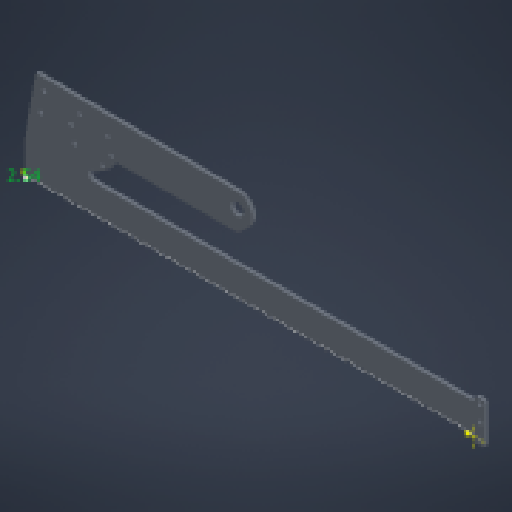
# Autodesk Inventor part: RACK_LINEARINTAKE
Saved by Autodesk Inventor 2026.2 (Build 302298010, 298A)
## iProperties
Created: 2026-04-01
Part Number: RACK_LINEARINTAKE
Material: Polycarbonate, RcM70, Black
Document SubType Name: Modeling
Designer: 4aida
Density: 11.9024 g/cm^3
Appearance: Grey (Dark)
Author: 4aida
Autodesk Inventor part; units mm, degrees
(part 1 of 2)
ref_plane "YZ Plane" through (0, 0, 0) normal (1, 0, 0) x (0, 1, 0)
ref_plane "XZ Plane" through (0, 0, 0) normal (0, 1, 0) x (-1, 0, 0)
ref_plane "XY Plane" through (0, 0, 0) normal (0, 0, 1) x (1, 0, 0)
sketch "Sketch1" plane through (0, 0, 0) normal (0, 0, 1) x (1, 0, 0)
  line L0 (7.1726, 5.588) -> (5.2604, 0.3343)
  arc A0 (4.783, 0) -> (5.2604, 0.3343) centre (4.783, 0.508) ccw
  line L1 (4.783, 0) -> (3.1966, 0)
  arc A1 (2.7192, 0.3343) -> (3.1966, 0) centre (3.1966, 0.508) ccw
  line L2 (2.7192, 0.3343) -> (0.807, 5.588)
  line L3 (-0.807, 5.588) -> (0.807, 5.588)
  line L4 (-0.807, 5.588) -> (-2.7192, 0.3343)
  arc A2 (-3.1966, 0) -> (-2.7192, 0.3343) centre (-3.1966, 0.508) ccw
  line L5 (-3.1966, 0) -> (-4.783, 0)
  arc A3 (-5.2604, 0.3343) -> (-4.783, 0) centre (-4.783, 0.508) ccw
  line L6 (-5.2604, 0.3343) -> (-7.1726, 5.588)
  line L7 (-3.9898, 0) -> (3.9898, 0) construction
  line L8 (7.1726, 27.5119) -> (7.1726, 38.1)
  line L9 (7.1726, 38.1) -> (-557.7681, 38.1)
  line L10 (-557.7681, 38.1) -> (-557.7681, 5.588)
  line L11 (-5.2604, 0.3343) -> (-7.1726, 5.588)
  line L12 (-11.9695, 0) -> (-3.9898, 0) construction
  line L13 (-8.7867, 5.588) -> (-10.6989, 0.3343)
  arc A4 (-11.1763, 0) -> (-10.6989, 0.3343) centre (-11.1763, 0.508) ccw
  line L14 (-11.1763, 0) -> (-12.7627, 0)
  arc A5 (-13.24, 0.3343) -> (-12.7627, 0) centre (-12.7627, 0.508) ccw
  line L15 (-13.24, 0.3343) -> (-15.1523, 5.588)
  arc A6 (-5.2604, 0.3343) -> (-4.783, 0) centre (-4.783, 0.508) ccw
  line L16 (-3.1966, 0) -> (-4.783, 0)
  arc A7 (-3.1966, 0) -> (-2.7192, 0.3343) centre (-3.1966, 0.508) ccw
  line L17 (-0.807, 5.588) -> (-2.7192, 0.3343)
  line L18 (-8.7867, 5.588) -> (-7.1726, 5.588)
  line L19 (-13.24, 0.3343) -> (-15.1523, 5.588)
  line L20 (-19.9491, 0) -> (-11.9695, 0) construction
  line L21 (-16.7663, 5.588) -> (-18.6785, 0.3343)
  arc A8 (-19.1559, 0) -> (-18.6785, 0.3343) centre (-19.1559, 0.508) ccw
  line L22 (-19.1559, 0) -> (-20.7423, 0)
  arc A9 (-21.2197, 0.3343) -> (-20.7423, 0) centre (-20.7423, 0.508) ccw
  line L23 (-21.2197, 0.3343) -> (-23.1319, 5.588)
  arc A10 (-13.24, 0.3343) -> (-12.7627, 0) centre (-12.7627, 0.508) ccw
  line L24 (-11.1763, 0) -> (-12.7627, 0)
  arc A11 (-11.1763, 0) -> (-10.6989, 0.3343) centre (-11.1763, 0.508) ccw
  line L25 (-8.7867, 5.588) -> (-10.6989, 0.3343)
  line L26 (-16.7663, 5.588) -> (-15.1523, 5.588)
  line L27 (-21.2197, 0.3343) -> (-23.1319, 5.588)
  line L28 (-27.9288, 0) -> (-19.9491, 0) construction
  line L29 (-24.746, 5.588) -> (-26.6582, 0.3343)
  arc A12 (-27.1355, 0) -> (-26.6582, 0.3343) centre (-27.1355, 0.508) ccw
  line L30 (-27.1355, 0) -> (-28.722, 0)
  arc A13 (-29.1993, 0.3343) -> (-28.722, 0) centre (-28.722, 0.508) ccw
  line L31 (-29.1993, 0.3343) -> (-31.1115, 5.588)
  arc A14 (-21.2197, 0.3343) -> (-20.7423, 0) centre (-20.7423, 0.508) ccw
  line L32 (-19.1559, 0) -> (-20.7423, 0)
  arc A15 (-19.1559, 0) -> (-18.6785, 0.3343) centre (-19.1559, 0.508) ccw
  line L33 (-16.7663, 5.588) -> (-18.6785, 0.3343)
  line L34 (-24.746, 5.588) -> (-23.1319, 5.588)
  line L35 (-29.1993, 0.3343) -> (-31.1115, 5.588)
  line L36 (-35.9084, 0) -> (-27.9288, 0) construction
  line L37 (-32.7256, 5.588) -> (-34.6378, 0.3343)
  arc A16 (-35.1152, 0) -> (-34.6378, 0.3343) centre (-35.1152, 0.508) ccw
  line L38 (-35.1152, 0) -> (-36.7016, 0)
  arc A17 (-37.179, 0.3343) -> (-36.7016, 0) centre (-36.7016, 0.508) ccw
  line L39 (-37.179, 0.3343) -> (-39.0912, 5.588)
  arc A18 (-29.1993, 0.3343) -> (-28.722, 0) centre (-28.722, 0.508) ccw
  line L40 (-27.1355, 0) -> (-28.722, 0)
  arc A19 (-27.1355, 0) -> (-26.6582, 0.3343) centre (-27.1355, 0.508) ccw
  line L41 (-24.746, 5.588) -> (-26.6582, 0.3343)
  line L42 (-32.7256, 5.588) -> (-31.1115, 5.588)
  line L43 (-37.179, 0.3343) -> (-39.0912, 5.588)
  line L44 (-43.888, 0) -> (-35.9084, 0) construction
  line L45 (-40.7053, 5.588) -> (-42.6175, 0.3343)
  arc A20 (-43.0948, 0) -> (-42.6175, 0.3343) centre (-43.0948, 0.508) ccw
  line L46 (-43.0948, 0) -> (-44.6813, 0)
  arc A21 (-45.1586, 0.3343) -> (-44.6813, 0) centre (-44.6813, 0.508) ccw
  line L47 (-45.1586, 0.3343) -> (-47.0708, 5.588)
  arc A22 (-37.179, 0.3343) -> (-36.7016, 0) centre (-36.7016, 0.508) ccw
  line L48 (-35.1152, 0) -> (-36.7016, 0)
  arc A23 (-35.1152, 0) -> (-34.6378, 0.3343) centre (-35.1152, 0.508) ccw
  line L49 (-32.7256, 5.588) -> (-34.6378, 0.3343)
  line L50 (-40.7053, 5.588) -> (-39.0912, 5.588)
  line L51 (-45.1586, 0.3343) -> (-47.0708, 5.588)
  line L52 (-51.8677, 0) -> (-43.888, 0) construction
  line L53 (-48.6849, 5.588) -> (-50.5971, 0.3343)
  arc A24 (-51.0745, 0) -> (-50.5971, 0.3343) centre (-51.0745, 0.508) ccw
  line L54 (-51.0745, 0) -> (-52.6609, 0)
  arc A25 (-53.1383, 0.3343) -> (-52.6609, 0) centre (-52.6609, 0.508) ccw
  line L55 (-53.1383, 0.3343) -> (-55.0505, 5.588)
  arc A26 (-45.1586, 0.3343) -> (-44.6813, 0) centre (-44.6813, 0.508) ccw
  line L56 (-43.0948, 0) -> (-44.6813, 0)
  arc A27 (-43.0948, 0) -> (-42.6175, 0.3343) centre (-43.0948, 0.508) ccw
  line L57 (-40.7053, 5.588) -> (-42.6175, 0.3343)
  line L58 (-48.6849, 5.588) -> (-47.0708, 5.588)
  line L59 (-53.1383, 0.3343) -> (-55.0505, 5.588)
  line L60 (-59.8473, 0) -> (-51.8677, 0) construction
  line L61 (-56.6646, 5.588) -> (-58.5768, 0.3343)
  arc A28 (-59.0541, 0) -> (-58.5768, 0.3343) centre (-59.0541, 0.508) ccw
  line L62 (-59.0541, 0) -> (-60.6406, 0)
  arc A29 (-61.1179, 0.3343) -> (-60.6406, 0) centre (-60.6406, 0.508) ccw
  line L63 (-61.1179, 0.3343) -> (-63.0301, 5.588)
  arc A30 (-53.1383, 0.3343) -> (-52.6609, 0) centre (-52.6609, 0.508) ccw
  line L64 (-51.0745, 0) -> (-52.6609, 0)
  arc A31 (-51.0745, 0) -> (-50.5971, 0.3343) centre (-51.0745, 0.508) ccw
  line L65 (-48.6849, 5.588) -> (-50.5971, 0.3343)
  line L66 (-56.6646, 5.588) -> (-55.0505, 5.588)
  line L67 (-61.1179, 0.3343) -> (-63.0301, 5.588)
  line L68 (-67.827, 0) -> (-59.8473, 0) construction
  line L69 (-64.6442, 5.588) -> (-66.5564, 0.3343)
  arc A32 (-67.0338, 0) -> (-66.5564, 0.3343) centre (-67.0338, 0.508) ccw
  line L70 (-67.0338, 0) -> (-68.6202, 0)
  arc A33 (-69.0976, 0.3343) -> (-68.6202, 0) centre (-68.6202, 0.508) ccw
  line L71 (-69.0976, 0.3343) -> (-71.0098, 5.588)
  arc A34 (-61.1179, 0.3343) -> (-60.6406, 0) centre (-60.6406, 0.508) ccw
  line L72 (-59.0541, 0) -> (-60.6406, 0)
  arc A35 (-59.0541, 0) -> (-58.5768, 0.3343) centre (-59.0541, 0.508) ccw
  line L73 (-56.6646, 5.588) -> (-58.5768, 0.3343)
  line L74 (-64.6442, 5.588) -> (-63.0301, 5.588)
  line L75 (-69.0976, 0.3343) -> (-71.0098, 5.588)
  line L76 (-75.8066, 0) -> (-67.827, 0) construction
  line L77 (-72.6238, 5.588) -> (-74.5361, 0.3343)
  arc A36 (-75.0134, 0) -> (-74.5361, 0.3343) centre (-75.0134, 0.508) ccw
  line L78 (-75.0134, 0) -> (-76.5998, 0)
  arc A37 (-77.0772, 0.3343) -> (-76.5998, 0) centre (-76.5998, 0.508) ccw
  line L79 (-77.0772, 0.3343) -> (-78.9894, 5.588)
  arc A38 (-69.0976, 0.3343) -> (-68.6202, 0) centre (-68.6202, 0.508) ccw
  line L80 (-67.0338, 0) -> (-68.6202, 0)
  arc A39 (-67.0338, 0) -> (-66.5564, 0.3343) centre (-67.0338, 0.508) ccw
  line L81 (-64.6442, 5.588) -> (-66.5564, 0.3343)
  line L82 (-72.6238, 5.588) -> (-71.0098, 5.588)
  line L83 (-77.0772, 0.3343) -> (-78.9894, 5.588)
  line L84 (-83.7863, 0) -> (-75.8066, 0) construction
  line L85 (-80.6035, 5.588) -> (-82.5157, 0.3343)
  arc A40 (-82.9931, 0) -> (-82.5157, 0.3343) centre (-82.9931, 0.508) ccw
  line L86 (-82.9931, 0) -> (-84.5795, 0)
  arc A41 (-85.0569, 0.3343) -> (-84.5795, 0) centre (-84.5795, 0.508) ccw
  line L87 (-85.0569, 0.3343) -> (-86.9691, 5.588)
  arc A42 (-77.0772, 0.3343) -> (-76.5998, 0) centre (-76.5998, 0.508) ccw
  line L88 (-75.0134, 0) -> (-76.5998, 0)
  arc A43 (-75.0134, 0) -> (-74.5361, 0.3343) centre (-75.0134, 0.508) ccw
  line L89 (-72.6238, 5.588) -> (-74.5361, 0.3343)
  line L90 (-80.6035, 5.588) -> (-78.9894, 5.588)
  line L91 (-85.0569, 0.3343) -> (-86.9691, 5.588)
  line L92 (-91.7659, 0) -> (-83.7863, 0) construction
  line L93 (-88.5831, 5.588) -> (-90.4953, 0.3343)
  arc A44 (-90.9727, 0) -> (-90.4953, 0.3343) centre (-90.9727, 0.508) ccw
  line L94 (-90.9727, 0) -> (-92.5591, 0)
  arc A45 (-93.0365, 0.3343) -> (-92.5591, 0) centre (-92.5591, 0.508) ccw
  line L95 (-93.0365, 0.3343) -> (-94.9487, 5.588)
  arc A46 (-85.0569, 0.3343) -> (-84.5795, 0) centre (-84.5795, 0.508) ccw
  line L96 (-82.9931, 0) -> (-84.5795, 0)
  arc A47 (-82.9931, 0) -> (-82.5157, 0.3343) centre (-82.9931, 0.508) ccw
  line L97 (-80.6035, 5.588) -> (-82.5157, 0.3343)
  line L98 (-88.5831, 5.588) -> (-86.9691, 5.588)
  line L99 (-93.0365, 0.3343) -> (-94.9487, 5.588)
  line L100 (-99.7456, 0) -> (-91.7659, 0) construction
  line L101 (-96.5628, 5.588) -> (-98.475, 0.3343)
  arc A48 (-98.9524, 0) -> (-98.475, 0.3343) centre (-98.9524, 0.508) ccw
  line L102 (-98.9524, 0) -> (-100.5388, 0)
  arc A49 (-101.0161, 0.3343) -> (-100.5388, 0) centre (-100.5388, 0.508) ccw
  line L103 (-101.0161, 0.3343) -> (-102.9284, 5.588)
  arc A50 (-93.0365, 0.3343) -> (-92.5591, 0) centre (-92.5591, 0.508) ccw
  line L104 (-90.9727, 0) -> (-92.5591, 0)
  arc A51 (-90.9727, 0) -> (-90.4953, 0.3343) centre (-90.9727, 0.508) ccw
  line L105 (-88.5831, 5.588) -> (-90.4953, 0.3343)
  line L106 (-96.5628, 5.588) -> (-94.9487, 5.588)
  line L107 (-101.0161, 0.3343) -> (-102.9284, 5.588)
  line L108 (-107.7252, 0) -> (-99.7456, 0) construction
  line L109 (-104.5424, 5.588) -> (-106.4546, 0.3343)
  arc A52 (-106.932, 0) -> (-106.4546, 0.3343) centre (-106.932, 0.508) ccw
  line L110 (-106.932, 0) -> (-108.5184, 0)
  arc A53 (-108.9958, 0.3343) -> (-108.5184, 0) centre (-108.5184, 0.508) ccw
  line L111 (-108.9958, 0.3343) -> (-110.908, 5.588)
  arc A54 (-101.0161, 0.3343) -> (-100.5388, 0) centre (-100.5388, 0.508) ccw
  line L112 (-98.9524, 0) -> (-100.5388, 0)
  arc A55 (-98.9524, 0) -> (-98.475, 0.3343) centre (-98.9524, 0.508) ccw
  line L113 (-96.5628, 5.588) -> (-98.475, 0.3343)
  line L114 (-104.5424, 5.588) -> (-102.9284, 5.588)
  line L115 (-108.9958, 0.3343) -> (-110.908, 5.588)
  line L116 (-115.7049, 0) -> (-107.7252, 0) construction
  line L117 (-112.5221, 5.588) -> (-114.4343, 0.3343)
  arc A56 (-114.9116, 0) -> (-114.4343, 0.3343) centre (-114.9116, 0.508) ccw
  line L118 (-114.9116, 0) -> (-116.4981, 0)
  arc A57 (-116.9754, 0.3343) -> (-116.4981, 0) centre (-116.4981, 0.508) ccw
  line L119 (-116.9754, 0.3343) -> (-118.8876, 5.588)
  arc A58 (-108.9958, 0.3343) -> (-108.5184, 0) centre (-108.5184, 0.508) ccw
  line L120 (-106.932, 0) -> (-108.5184, 0)
  arc A59 (-106.932, 0) -> (-106.4546, 0.3343) centre (-106.932, 0.508) ccw
  line L121 (-104.5424, 5.588) -> (-106.4546, 0.3343)
  line L122 (-112.5221, 5.588) -> (-110.908, 5.588)
  line L123 (-116.9754, 0.3343) -> (-118.8876, 5.588)
  line L124 (-123.6845, 0) -> (-115.7049, 0) construction
  line L125 (-120.5017, 5.588) -> (-122.4139, 0.3343)
  arc A60 (-122.8913, 0) -> (-122.4139, 0.3343) centre (-122.8913, 0.508) ccw
  line L126 (-122.8913, 0) -> (-124.4777, 0)
  arc A61 (-124.9551, 0.3343) -> (-124.4777, 0) centre (-124.4777, 0.508) ccw
  line L127 (-124.9551, 0.3343) -> (-126.8673, 5.588)
  arc A62 (-116.9754, 0.3343) -> (-116.4981, 0) centre (-116.4981, 0.508) ccw
  line L128 (-114.9116, 0) -> (-116.4981, 0)
  arc A63 (-114.9116, 0) -> (-114.4343, 0.3343) centre (-114.9116, 0.508) ccw
  line L129 (-112.5221, 5.588) -> (-114.4343, 0.3343)
  line L130 (-120.5017, 5.588) -> (-118.8876, 5.588)
  line L131 (-124.9551, 0.3343) -> (-126.8673, 5.588)
  line L132 (-131.6641, 0) -> (-123.6845, 0) construction
  line L133 (-128.4814, 5.588) -> (-130.3936, 0.3343)
  arc A64 (-130.8709, 0) -> (-130.3936, 0.3343) centre (-130.8709, 0.508) ccw
  line L134 (-130.8709, 0) -> (-132.4574, 0)
  arc A65 (-132.9347, 0.3343) -> (-132.4574, 0) centre (-132.4574, 0.508) ccw
  line L135 (-132.9347, 0.3343) -> (-134.8469, 5.588)
  arc A66 (-124.9551, 0.3343) -> (-124.4777, 0) centre (-124.4777, 0.508) ccw
  line L136 (-122.8913, 0) -> (-124.4777, 0)
  arc A67 (-122.8913, 0) -> (-122.4139, 0.3343) centre (-122.8913, 0.508) ccw
  line L137 (-120.5017, 5.588) -> (-122.4139, 0.3343)
  line L138 (-128.4814, 5.588) -> (-126.8673, 5.588)
  line L139 (-132.9347, 0.3343) -> (-134.8469, 5.588)
  line L140 (-139.6438, 0) -> (-131.6641, 0) construction
  line L141 (-136.461, 5.588) -> (-138.3732, 0.3343)
  arc A68 (-138.8506, 0) -> (-138.3732, 0.3343) centre (-138.8506, 0.508) ccw
  line L142 (-138.8506, 0) -> (-140.437, 0)
  arc A69 (-140.9144, 0.3343) -> (-140.437, 0) centre (-140.437, 0.508) ccw
  line L143 (-140.9144, 0.3343) -> (-142.8266, 5.588)
  arc A70 (-132.9347, 0.3343) -> (-132.4574, 0) centre (-132.4574, 0.508) ccw
  line L144 (-130.8709, 0) -> (-132.4574, 0)
  arc A71 (-130.8709, 0) -> (-130.3936, 0.3343) centre (-130.8709, 0.508) ccw
  line L145 (-128.4814, 5.588) -> (-130.3936, 0.3343)
  line L146 (-136.461, 5.588) -> (-134.8469, 5.588)
  line L147 (-140.9144, 0.3343) -> (-142.8266, 5.588)
  line L148 (-147.6234, 0) -> (-139.6438, 0) construction
  line L149 (-144.4407, 5.588) -> (-146.3529, 0.3343)
  arc A72 (-146.8302, 0) -> (-146.3529, 0.3343) centre (-146.8302, 0.508) ccw
  line L150 (-146.8302, 0) -> (-148.4167, 0)
  arc A73 (-148.894, 0.3343) -> (-148.4167, 0) centre (-148.4167, 0.508) ccw
  line L151 (-148.894, 0.3343) -> (-150.8062, 5.588)
  arc A74 (-140.9144, 0.3343) -> (-140.437, 0) centre (-140.437, 0.508) ccw
  line L152 (-138.8506, 0) -> (-140.437, 0)
  arc A75 (-138.8506, 0) -> (-138.3732, 0.3343) centre (-138.8506, 0.508) ccw
  line L153 (-136.461, 5.588) -> (-138.3732, 0.3343)
  line L154 (-144.4407, 5.588) -> (-142.8266, 5.588)
  line L155 (-148.894, 0.3343) -> (-150.8062, 5.588)
  line L156 (-155.6031, 0) -> (-147.6234, 0) construction
  line L157 (-152.4203, 5.588) -> (-154.3325, 0.3343)
  arc A76 (-154.8099, 0) -> (-154.3325, 0.3343) centre (-154.8099, 0.508) ccw
  line L158 (-154.8099, 0) -> (-156.3963, 0)
  arc A77 (-156.8737, 0.3343) -> (-156.3963, 0) centre (-156.3963, 0.508) ccw
  line L159 (-156.8737, 0.3343) -> (-158.7859, 5.588)
  arc A78 (-148.894, 0.3343) -> (-148.4167, 0) centre (-148.4167, 0.508) ccw
  line L160 (-146.8302, 0) -> (-148.4167, 0)
  arc A79 (-146.8302, 0) -> (-146.3529, 0.3343) centre (-146.8302, 0.508) ccw
  line L161 (-144.4407, 5.588) -> (-146.3529, 0.3343)
  line L162 (-152.4203, 5.588) -> (-150.8062, 5.588)
  line L163 (-156.8737, 0.3343) -> (-158.7859, 5.588)
  line L164 (-163.5827, 0) -> (-155.6031, 0) construction
  line L165 (-160.3999, 5.588) -> (-162.3122, 0.3343)
  arc A80 (-162.7895, 0) -> (-162.3122, 0.3343) centre (-162.7895, 0.508) ccw
  line L166 (-162.7895, 0) -> (-164.3759, 0)
  arc A81 (-164.8533, 0.3343) -> (-164.3759, 0) centre (-164.3759, 0.508) ccw
  line L167 (-164.8533, 0.3343) -> (-166.7655, 5.588)
  arc A82 (-156.8737, 0.3343) -> (-156.3963, 0) centre (-156.3963, 0.508) ccw
  line L168 (-154.8099, 0) -> (-156.3963, 0)
  arc A83 (-154.8099, 0) -> (-154.3325, 0.3343) centre (-154.8099, 0.508) ccw
  line L169 (-152.4203, 5.588) -> (-154.3325, 0.3343)
  line L170 (-160.3999, 5.588) -> (-158.7859, 5.588)
  line L171 (-164.8533, 0.3343) -> (-166.7655, 5.588)
  line L172 (-171.5624, 0) -> (-163.5827, 0) construction
  line L173 (-168.3796, 5.588) -> (-170.2918, 0.3343)
  arc A84 (-170.7692, 0) -> (-170.2918, 0.3343) centre (-170.7692, 0.508) ccw
  line L174 (-170.7692, 0) -> (-172.3556, 0)
  arc A85 (-172.833, 0.3343) -> (-172.3556, 0) centre (-172.3556, 0.508) ccw
  line L175 (-172.833, 0.3343) -> (-174.7452, 5.588)
  arc A86 (-164.8533, 0.3343) -> (-164.3759, 0) centre (-164.3759, 0.508) ccw
  line L176 (-162.7895, 0) -> (-164.3759, 0)
  arc A87 (-162.7895, 0) -> (-162.3122, 0.3343) centre (-162.7895, 0.508) ccw
  line L177 (-160.3999, 5.588) -> (-162.3122, 0.3343)
  line L178 (-168.3796, 5.588) -> (-166.7655, 5.588)
  line L179 (-172.833, 0.3343) -> (-174.7452, 5.588)
  line L180 (-179.542, 0) -> (-171.5624, 0) construction
  line L181 (-176.3592, 5.588) -> (-178.2714, 0.3343)
  arc A88 (-178.7488, 0) -> (-178.2714, 0.3343) centre (-178.7488, 0.508) ccw
  line L182 (-178.7488, 0) -> (-180.3352, 0)
  arc A89 (-180.8126, 0.3343) -> (-180.3352, 0) centre (-180.3352, 0.508) ccw
  line L183 (-180.8126, 0.3343) -> (-182.7248, 5.588)
  arc A90 (-172.833, 0.3343) -> (-172.3556, 0) centre (-172.3556, 0.508) ccw
  line L184 (-170.7692, 0) -> (-172.3556, 0)
  arc A91 (-170.7692, 0) -> (-170.2918, 0.3343) centre (-170.7692, 0.508) ccw
  line L185 (-168.3796, 5.588) -> (-170.2918, 0.3343)
  line L186 (-176.3592, 5.588) -> (-174.7452, 5.588)
  line L187 (-180.8126, 0.3343) -> (-182.7248, 5.588)
  line L188 (-187.5217, 0) -> (-179.542, 0) construction
  line L189 (-184.3389, 5.588) -> (-186.2511, 0.3343)
  arc A92 (-186.7285, 0) -> (-186.2511, 0.3343) centre (-186.7285, 0.508) ccw
  line L190 (-186.7285, 0) -> (-188.3149, 0)
  arc A93 (-188.7922, 0.3343) -> (-188.3149, 0) centre (-188.3149, 0.508) ccw
  line L191 (-188.7922, 0.3343) -> (-190.7044, 5.588)
  arc A94 (-180.8126, 0.3343) -> (-180.3352, 0) centre (-180.3352, 0.508) ccw
  line L192 (-178.7488, 0) -> (-180.3352, 0)
  arc A95 (-178.7488, 0) -> (-178.2714, 0.3343) centre (-178.7488, 0.508) ccw
  line L193 (-176.3592, 5.588) -> (-178.2714, 0.3343)
  line L194 (-184.3389, 5.588) -> (-182.7248, 5.588)
  line L195 (-188.7922, 0.3343) -> (-190.7044, 5.588)
  line L196 (-195.5013, 0) -> (-187.5217, 0) construction
  line L197 (-192.3185, 5.588) -> (-194.2307, 0.3343)
  arc A96 (-194.7081, 0) -> (-194.2307, 0.3343) centre (-194.7081, 0.508) ccw
  line L198 (-194.7081, 0) -> (-196.2945, 0)
  arc A97 (-196.7719, 0.3343) -> (-196.2945, 0) centre (-196.2945, 0.508) ccw
  line L199 (-196.7719, 0.3343) -> (-198.6841, 5.588)
  arc A98 (-188.7922, 0.3343) -> (-188.3149, 0) centre (-188.3149, 0.508) ccw
  line L200 (-186.7285, 0) -> (-188.3149, 0)
  arc A99 (-186.7285, 0) -> (-186.2511, 0.3343) centre (-186.7285, 0.508) ccw
  line L201 (-184.3389, 5.588) -> (-186.2511, 0.3343)
  line L202 (-192.3185, 5.588) -> (-190.7044, 5.588)
  line L203 (-196.7719, 0.3343) -> (-198.6841, 5.588)
  line L204 (-203.481, 0) -> (-195.5013, 0) construction
  line L205 (-200.2982, 5.588) -> (-202.2104, 0.3343)
  arc A100 (-202.6877, 0) -> (-202.2104, 0.3343) centre (-202.6877, 0.508) ccw
  line L206 (-202.6877, 0) -> (-204.2742, 0)
  arc A101 (-204.7515, 0.3343) -> (-204.2742, 0) centre (-204.2742, 0.508) ccw
  line L207 (-204.7515, 0.3343) -> (-206.6637, 5.588)
  arc A102 (-196.7719, 0.3343) -> (-196.2945, 0) centre (-196.2945, 0.508) ccw
  line L208 (-194.7081, 0) -> (-196.2945, 0)
  arc A103 (-194.7081, 0) -> (-194.2307, 0.3343) centre (-194.7081, 0.508) ccw
  line L209 (-192.3185, 5.588) -> (-194.2307, 0.3343)
  line L210 (-200.2982, 5.588) -> (-198.6841, 5.588)
  line L211 (-204.7515, 0.3343) -> (-206.6637, 5.588)
  line L212 (-211.4606, 0) -> (-203.481, 0) construction
  line L213 (-208.2778, 5.588) -> (-210.19, 0.3343)
  arc A104 (-210.6674, 0) -> (-210.19, 0.3343) centre (-210.6674, 0.508) ccw
  line L214 (-210.6674, 0) -> (-212.2538, 0)
  arc A105 (-212.7312, 0.3343) -> (-212.2538, 0) centre (-212.2538, 0.508) ccw
  line L215 (-212.7312, 0.3343) -> (-214.6434, 5.588)
  arc A106 (-204.7515, 0.3343) -> (-204.2742, 0) centre (-204.2742, 0.508) ccw
  line L216 (-202.6877, 0) -> (-204.2742, 0)
  arc A107 (-202.6877, 0) -> (-202.2104, 0.3343) centre (-202.6877, 0.508) ccw
  line L217 (-200.2982, 5.588) -> (-202.2104, 0.3343)
  line L218 (-208.2778, 5.588) -> (-206.6637, 5.588)
  line L219 (-212.7312, 0.3343) -> (-214.6434, 5.588)
  line L220 (-219.4402, 0) -> (-211.4606, 0) construction
  line L221 (-216.2575, 5.588) -> (-218.1697, 0.3343)
  arc A108 (-218.647, 0) -> (-218.1697, 0.3343) centre (-218.647, 0.508) ccw
  line L222 (-218.647, 0) -> (-220.2335, 0)
  arc A109 (-220.7108, 0.3343) -> (-220.2335, 0) centre (-220.2335, 0.508) ccw
  line L223 (-220.7108, 0.3343) -> (-222.623, 5.588)
  arc A110 (-212.7312, 0.3343) -> (-212.2538, 0) centre (-212.2538, 0.508) ccw
  line L224 (-210.6674, 0) -> (-212.2538, 0)
  arc A111 (-210.6674, 0) -> (-210.19, 0.3343) centre (-210.6674, 0.508) ccw
  line L225 (-208.2778, 5.588) -> (-210.19, 0.3343)
  line L226 (-216.2575, 5.588) -> (-214.6434, 5.588)
  line L227 (-220.7108, 0.3343) -> (-222.623, 5.588)
  line L228 (-227.4199, 0) -> (-219.4402, 0) construction
  line L229 (-224.2371, 5.588) -> (-226.1493, 0.3343)
  arc A112 (-226.6267, 0) -> (-226.1493, 0.3343) centre (-226.6267, 0.508) ccw
  line L230 (-226.6267, 0) -> (-228.2131, 0)
  arc A113 (-228.6905, 0.3343) -> (-228.2131, 0) centre (-228.2131, 0.508) ccw
  line L231 (-228.6905, 0.3343) -> (-230.6027, 5.588)
  arc A114 (-220.7108, 0.3343) -> (-220.2335, 0) centre (-220.2335, 0.508) ccw
  line L232 (-218.647, 0) -> (-220.2335, 0)
  arc A115 (-218.647, 0) -> (-218.1697, 0.3343) centre (-218.647, 0.508) ccw
  line L233 (-216.2575, 5.588) -> (-218.1697, 0.3343)
  line L234 (-224.2371, 5.588) -> (-222.623, 5.588)
  line L235 (-228.6905, 0.3343) -> (-230.6027, 5.588)
  line L236 (-235.3995, 0) -> (-227.4199, 0) construction
  line L237 (-232.2168, 5.588) -> (-234.129, 0.3343)
  arc A116 (-234.6063, 0) -> (-234.129, 0.3343) centre (-234.6063, 0.508) ccw
  line L238 (-234.6063, 0) -> (-236.1928, 0)
  arc A117 (-236.6701, 0.3343) -> (-236.1928, 0) centre (-236.1928, 0.508) ccw
  line L239 (-236.6701, 0.3343) -> (-238.5823, 5.588)
  arc A118 (-228.6905, 0.3343) -> (-228.2131, 0) centre (-228.2131, 0.508) ccw
  line L240 (-226.6267, 0) -> (-228.2131, 0)
  arc A119 (-226.6267, 0) -> (-226.1493, 0.3343) centre (-226.6267, 0.508) ccw
  line L241 (-224.2371, 5.588) -> (-226.1493, 0.3343)
  line L242 (-232.2168, 5.588) -> (-230.6027, 5.588)
  line L243 (-236.6701, 0.3343) -> (-238.5823, 5.588)
  line L244 (-243.3792, 0) -> (-235.3995, 0) construction
  line L245 (-240.1964, 5.588) -> (-242.1086, 0.3343)
  arc A120 (-242.586, 0) -> (-242.1086, 0.3343) centre (-242.586, 0.508) ccw
  line L246 (-242.586, 0) -> (-244.1724, 0)
  arc A121 (-244.6498, 0.3343) -> (-244.1724, 0) centre (-244.1724, 0.508) ccw
  line L247 (-244.6498, 0.3343) -> (-246.562, 5.588)
  arc A122 (-236.6701, 0.3343) -> (-236.1928, 0) centre (-236.1928, 0.508) ccw
  line L248 (-234.6063, 0) -> (-236.1928, 0)
  arc A123 (-234.6063, 0) -> (-234.129, 0.3343) centre (-234.6063, 0.508) ccw
  line L249 (-232.2168, 5.588) -> (-234.129, 0.3343)
  line L250 (-240.1964, 5.588) -> (-238.5823, 5.588)
  line L251 (-244.6498, 0.3343) -> (-246.562, 5.588)
  line L252 (-251.3588, 0) -> (-243.3792, 0) construction
  line L253 (-248.176, 5.588) -> (-250.0883, 0.3343)
  arc A124 (-250.5656, 0) -> (-250.0883, 0.3343) centre (-250.5656, 0.508) ccw
  line L254 (-250.5656, 0) -> (-252.152, 0)
  arc A125 (-252.6294, 0.3343) -> (-252.152, 0) centre (-252.152, 0.508) ccw
  line L255 (-252.6294, 0.3343) -> (-254.5416, 5.588)
  arc A126 (-244.6498, 0.3343) -> (-244.1724, 0) centre (-244.1724, 0.508) ccw
  line L256 (-242.586, 0) -> (-244.1724, 0)
  arc A127 (-242.586, 0) -> (-242.1086, 0.3343) centre (-242.586, 0.508) ccw
  line L257 (-240.1964, 5.588) -> (-242.1086, 0.3343)
  line L258 (-248.176, 5.588) -> (-246.562, 5.588)
  line L259 (-252.6294, 0.3343) -> (-254.5416, 5.588)
  line L260 (-259.3385, 0) -> (-251.3588, 0) construction
  line L261 (-256.1557, 5.588) -> (-258.0679, 0.3343)
  arc A128 (-258.5453, 0) -> (-258.0679, 0.3343) centre (-258.5453, 0.508) ccw
  line L262 (-258.5453, 0) -> (-260.1317, 0)
  arc A129 (-260.6091, 0.3343) -> (-260.1317, 0) centre (-260.1317, 0.508) ccw
  line L263 (-260.6091, 0.3343) -> (-262.5213, 5.588)
  arc A130 (-252.6294, 0.3343) -> (-252.152, 0) centre (-252.152, 0.508) ccw
  line L264 (-250.5656, 0) -> (-252.152, 0)
  arc A131 (-250.5656, 0) -> (-250.0883, 0.3343) centre (-250.5656, 0.508) ccw
  line L265 (-248.176, 5.588) -> (-250.0883, 0.3343)
  line L266 (-256.1557, 5.588) -> (-254.5416, 5.588)
  line L267 (-260.6091, 0.3343) -> (-262.5213, 5.588)
  line L268 (-267.3181, 0) -> (-259.3385, 0) construction
  line L269 (-264.1353, 5.588) -> (-266.0475, 0.3343)
  arc A132 (-266.5249, 0) -> (-266.0475, 0.3343) centre (-266.5249, 0.508) ccw
  line L270 (-266.5249, 0) -> (-268.1113, 0)
  arc A133 (-268.5887, 0.3343) -> (-268.1113, 0) centre (-268.1113, 0.508) ccw
  line L271 (-268.5887, 0.3343) -> (-270.5009, 5.588)
  arc A134 (-260.6091, 0.3343) -> (-260.1317, 0) centre (-260.1317, 0.508) ccw
  line L272 (-258.5453, 0) -> (-260.1317, 0)
  arc A135 (-258.5453, 0) -> (-258.0679, 0.3343) centre (-258.5453, 0.508) ccw
  line L273 (-256.1557, 5.588) -> (-258.0679, 0.3343)
  line L274 (-264.1353, 5.588) -> (-262.5213, 5.588)
  line L275 (-268.5887, 0.3343) -> (-270.5009, 5.588)
  line L276 (-275.2978, 0) -> (-267.3181, 0) construction
  line L277 (-272.115, 5.588) -> (-274.0272, 0.3343)
  arc A136 (-274.5046, 0) -> (-274.0272, 0.3343) centre (-274.5046, 0.508) ccw
  line L278 (-274.5046, 0) -> (-276.091, 0)
  arc A137 (-276.5683, 0.3343) -> (-276.091, 0) centre (-276.091, 0.508) ccw
  line L279 (-276.5683, 0.3343) -> (-278.4805, 5.588)
  arc A138 (-268.5887, 0.3343) -> (-268.1113, 0) centre (-268.1113, 0.508) ccw
  line L280 (-266.5249, 0) -> (-268.1113, 0)
  arc A139 (-266.5249, 0) -> (-266.0475, 0.3343) centre (-266.5249, 0.508) ccw
  line L281 (-264.1353, 5.588) -> (-266.0475, 0.3343)
  line L282 (-272.115, 5.588) -> (-270.5009, 5.588)
  line L283 (-276.5683, 0.3343) -> (-278.4805, 5.588)
  line L284 (-283.2774, 0) -> (-275.2978, 0) construction
  line L285 (-280.0946, 5.588) -> (-282.0068, 0.3343)
  arc A140 (-282.4842, 0) -> (-282.0068, 0.3343) centre (-282.4842, 0.508) ccw
  line L286 (-282.4842, 0) -> (-284.0706, 0)
  arc A141 (-284.548, 0.3343) -> (-284.0706, 0) centre (-284.0706, 0.508) ccw
  line L287 (-284.548, 0.3343) -> (-286.4602, 5.588)
  arc A142 (-276.5683, 0.3343) -> (-276.091, 0) centre (-276.091, 0.508) ccw
  line L288 (-274.5046, 0) -> (-276.091, 0)
  arc A143 (-274.5046, 0) -> (-274.0272, 0.3343) centre (-274.5046, 0.508) ccw
  line L289 (-272.115, 5.588) -> (-274.0272, 0.3343)
  line L290 (-280.0946, 5.588) -> (-278.4805, 5.588)
  line L291 (-284.548, 0.3343) -> (-286.4602, 5.588)
  line L292 (-291.2571, 0) -> (-283.2774, 0) construction
  line L293 (-288.0743, 5.588) -> (-289.9865, 0.3343)
  arc A144 (-290.4638, 0) -> (-289.9865, 0.3343) centre (-290.4638, 0.508) ccw
  line L294 (-290.4638, 0) -> (-292.0503, 0)
  arc A145 (-292.5276, 0.3343) -> (-292.0503, 0) centre (-292.0503, 0.508) ccw
  line L295 (-292.5276, 0.3343) -> (-294.4398, 5.588)
  arc A146 (-284.548, 0.3343) -> (-284.0706, 0) centre (-284.0706, 0.508) ccw
  line L296 (-282.4842, 0) -> (-284.0706, 0)
  arc A147 (-282.4842, 0) -> (-282.0068, 0.3343) centre (-282.4842, 0.508) ccw
  line L297 (-280.0946, 5.588) -> (-282.0068, 0.3343)
  line L298 (-288.0743, 5.588) -> (-286.4602, 5.588)
  line L299 (-292.5276, 0.3343) -> (-294.4398, 5.588)
  line L300 (-299.2367, 0) -> (-291.2571, 0) construction
  line L301 (-296.0539, 5.588) -> (-297.9661, 0.3343)
  arc A148 (-298.4435, 0) -> (-297.9661, 0.3343) centre (-298.4435, 0.508) ccw
  line L302 (-298.4435, 0) -> (-300.0299, 0)
  arc A149 (-300.5073, 0.3343) -> (-300.0299, 0) centre (-300.0299, 0.508) ccw
  line L303 (-300.5073, 0.3343) -> (-302.4195, 5.588)
  arc A150 (-292.5276, 0.3343) -> (-292.0503, 0) centre (-292.0503, 0.508) ccw
  line L304 (-290.4638, 0) -> (-292.0503, 0)
  arc A151 (-290.4638, 0) -> (-289.9865, 0.3343) centre (-290.4638, 0.508) ccw
  line L305 (-288.0743, 5.588) -> (-289.9865, 0.3343)
  line L306 (-296.0539, 5.588) -> (-294.4398, 5.588)
  line L307 (-300.5073, 0.3343) -> (-302.4195, 5.588)
  line L308 (-307.2163, 0) -> (-299.2367, 0) construction
  line L309 (-304.0336, 5.588) -> (-305.9458, 0.3343)
  arc A152 (-306.4231, 0) -> (-305.9458, 0.3343) centre (-306.4231, 0.508) ccw
  line L310 (-306.4231, 0) -> (-308.0096, 0)
  arc A153 (-308.4869, 0.3343) -> (-308.0096, 0) centre (-308.0096, 0.508) ccw
  line L311 (-308.4869, 0.3343) -> (-310.3991, 5.588)
  arc A154 (-300.5073, 0.3343) -> (-300.0299, 0) centre (-300.0299, 0.508) ccw
  line L312 (-298.4435, 0) -> (-300.0299, 0)
  arc A155 (-298.4435, 0) -> (-297.9661, 0.3343) centre (-298.4435, 0.508) ccw
  line L313 (-296.0539, 5.588) -> (-297.9661, 0.3343)
  line L314 (-304.0336, 5.588) -> (-302.4195, 5.588)
  line L315 (-308.4869, 0.3343) -> (-310.3991, 5.588)
  line L316 (-315.196, 0) -> (-307.2163, 0) construction
  line L317 (-312.0132, 5.588) -> (-313.9254, 0.3343)
  arc A156 (-314.4028, 0) -> (-313.9254, 0.3343) centre (-314.4028, 0.508) ccw
  line L318 (-314.4028, 0) -> (-315.9892, 0)
  arc A157 (-316.4666, 0.3343) -> (-315.9892, 0) centre (-315.9892, 0.508) ccw
  line L319 (-316.4666, 0.3343) -> (-318.3788, 5.588)
  arc A158 (-308.4869, 0.3343) -> (-308.0096, 0) centre (-308.0096, 0.508) ccw
  line L320 (-306.4231, 0) -> (-308.0096, 0)
  arc A159 (-306.4231, 0) -> (-305.9458, 0.3343) centre (-306.4231, 0.508) ccw
  line L321 (-304.0336, 5.588) -> (-305.9458, 0.3343)
  line L322 (-312.0132, 5.588) -> (-310.3991, 5.588)
  line L323 (-316.4666, 0.3343) -> (-318.3788, 5.588)
  line L324 (-323.1756, 0) -> (-315.196, 0) construction
  line L325 (-319.9929, 5.588) -> (-321.9051, 0.3343)
  arc A160 (-322.3824, 0) -> (-321.9051, 0.3343) centre (-322.3824, 0.508) ccw
  line L326 (-322.3824, 0) -> (-323.9688, 0)
  arc A161 (-324.4462, 0.3343) -> (-323.9688, 0) centre (-323.9688, 0.508) ccw
  line L327 (-324.4462, 0.3343) -> (-326.3584, 5.588)
  arc A162 (-316.4666, 0.3343) -> (-315.9892, 0) centre (-315.9892, 0.508) ccw
  line L328 (-314.4028, 0) -> (-315.9892, 0)
  arc A163 (-314.4028, 0) -> (-313.9254, 0.3343) centre (-314.4028, 0.508) ccw
  line L329 (-312.0132, 5.588) -> (-313.9254, 0.3343)
  line L330 (-319.9929, 5.588) -> (-318.3788, 5.588)
  line L331 (-324.4462, 0.3343) -> (-326.3584, 5.588)
  line L332 (-331.1553, 0) -> (-323.1756, 0) construction
  line L333 (-327.9725, 5.588) -> (-329.8847, 0.3343)
  arc A164 (-330.3621, 0) -> (-329.8847, 0.3343) centre (-330.3621, 0.508) ccw
  line L334 (-330.3621, 0) -> (-331.9485, 0)
  arc A165 (-332.4259, 0.3343) -> (-331.9485, 0) centre (-331.9485, 0.508) ccw
  line L335 (-332.4259, 0.3343) -> (-334.3381, 5.588)
  arc A166 (-324.4462, 0.3343) -> (-323.9688, 0) centre (-323.9688, 0.508) ccw
  line L336 (-322.3824, 0) -> (-323.9688, 0)
  arc A167 (-322.3824, 0) -> (-321.9051, 0.3343) centre (-322.3824, 0.508) ccw
  line L337 (-319.9929, 5.588) -> (-321.9051, 0.3343)
  line L338 (-327.9725, 5.588) -> (-326.3584, 5.588)
  line L339 (-332.4259, 0.3343) -> (-334.3381, 5.588)
  line L340 (-339.1349, 0) -> (-331.1553, 0) construction
  line L341 (-335.9521, 5.588) -> (-337.8644, 0.3343)
  arc A168 (-338.3417, 0) -> (-337.8644, 0.3343) centre (-338.3417, 0.508) ccw
  line L342 (-338.3417, 0) -> (-339.9281, 0)
  arc A169 (-340.4055, 0.3343) -> (-339.9281, 0) centre (-339.9281, 0.508) ccw
  line L343 (-340.4055, 0.3343) -> (-342.3177, 5.588)
  arc A170 (-332.4259, 0.3343) -> (-331.9485, 0) centre (-331.9485, 0.508) ccw
  line L344 (-330.3621, 0) -> (-331.9485, 0)
  arc A171 (-330.3621, 0) -> (-329.8847, 0.3343) centre (-330.3621, 0.508) ccw
  line L345 (-327.9725, 5.588) -> (-329.8847, 0.3343)
  line L346 (-335.9521, 5.588) -> (-334.3381, 5.588)
  line L347 (-340.4055, 0.3343) -> (-342.3177, 5.588)
  line L348 (-347.1146, 0) -> (-339.1349, 0) construction
  line L349 (-343.9318, 5.588) -> (-345.844, 0.3343)
  arc A172 (-346.3214, 0) -> (-345.844, 0.3343) centre (-346.3214, 0.508) ccw
  line L350 (-346.3214, 0) -> (-347.9078, 0)
  arc A173 (-348.3851, 0.3343) -> (-347.9078, 0) centre (-347.9078, 0.508) ccw
  line L351 (-348.3851, 0.3343) -> (-350.2974, 5.588)
  arc A174 (-340.4055, 0.3343) -> (-339.9281, 0) centre (-339.9281, 0.508) ccw
  line L352 (-338.3417, 0) -> (-339.9281, 0)
  arc A175 (-338.3417, 0) -> (-337.8644, 0.3343) centre (-338.3417, 0.508) ccw
  line L353 (-335.9521, 5.588) -> (-337.8644, 0.3343)
  line L354 (-343.9318, 5.588) -> (-342.3177, 5.588)
  line L355 (-348.3851, 0.3343) -> (-350.2974, 5.588)
  line L356 (-355.0942, 0) -> (-347.1146, 0) construction
  line L357 (-351.9114, 5.588) -> (-353.8236, 0.3343)
  arc A176 (-354.301, 0) -> (-353.8236, 0.3343) centre (-354.301, 0.508) ccw
  line L358 (-354.301, 0) -> (-355.8874, 0)
  arc A177 (-356.3648, 0.3343) -> (-355.8874, 0) centre (-355.8874, 0.508) ccw
  line L359 (-356.3648, 0.3343) -> (-358.277, 5.588)
  arc A178 (-348.3851, 0.3343) -> (-347.9078, 0) centre (-347.9078, 0.508) ccw
  line L360 (-346.3214, 0) -> (-347.9078, 0)
  arc A179 (-346.3214, 0) -> (-345.844, 0.3343) centre (-346.3214, 0.508) ccw
  line L361 (-343.9318, 5.588) -> (-345.844, 0.3343)
  line L362 (-351.9114, 5.588) -> (-350.2974, 5.588)
  line L363 (-356.3648, 0.3343) -> (-358.277, 5.588)
  line L364 (-363.0739, 0) -> (-355.0942, 0) construction
  line L365 (-359.8911, 5.588) -> (-361.8033, 0.3343)
  arc A180 (-362.2806, 0) -> (-361.8033, 0.3343) centre (-362.2806, 0.508) ccw
  line L366 (-362.2806, 0) -> (-363.8671, 0)
  arc A181 (-364.3444, 0.3343) -> (-363.8671, 0) centre (-363.8671, 0.508) ccw
  line L367 (-364.3444, 0.3343) -> (-366.2566, 5.588)
  arc A182 (-356.3648, 0.3343) -> (-355.8874, 0) centre (-355.8874, 0.508) ccw
  line L368 (-354.301, 0) -> (-355.8874, 0)
  arc A183 (-354.301, 0) -> (-353.8236, 0.3343) centre (-354.301, 0.508) ccw
  line L369 (-351.9114, 5.588) -> (-353.8236, 0.3343)
  line L370 (-359.8911, 5.588) -> (-358.277, 5.588)
  line L371 (-364.3444, 0.3343) -> (-366.2566, 5.588)
  line L372 (-371.0535, 0) -> (-363.0739, 0) construction
  line L373 (-367.8707, 5.588) -> (-369.7829, 0.3343)
  arc A184 (-370.2603, 0) -> (-369.7829, 0.3343) centre (-370.2603, 0.508) ccw
  line L374 (-370.2603, 0) -> (-371.8467, 0)
  arc A185 (-372.3241, 0.3343) -> (-371.8467, 0) centre (-371.8467, 0.508) ccw
  line L375 (-372.3241, 0.3343) -> (-374.2363, 5.588)
  arc A186 (-364.3444, 0.3343) -> (-363.8671, 0) centre (-363.8671, 0.508) ccw
  line L376 (-362.2806, 0) -> (-363.8671, 0)
  arc A187 (-362.2806, 0) -> (-361.8033, 0.3343) centre (-362.2806, 0.508) ccw
  line L377 (-359.8911, 5.588) -> (-361.8033, 0.3343)
  line L378 (-367.8707, 5.588) -> (-366.2566, 5.588)
  line L379 (-372.3241, 0.3343) -> (-374.2363, 5.588)
  line L380 (-379.0332, 0) -> (-371.0535, 0) construction
  line L381 (-375.8504, 5.588) -> (-377.7626, 0.3343)
  arc A188 (-378.2399, 0) -> (-377.7626, 0.3343) centre (-378.2399, 0.508) ccw
  line L382 (-378.2399, 0) -> (-379.8264, 0)
  arc A189 (-380.3037, 0.3343) -> (-379.8264, 0) centre (-379.8264, 0.508) ccw
  line L383 (-380.3037, 0.3343) -> (-382.2159, 5.588)
  arc A190 (-372.3241, 0.3343) -> (-371.8467, 0) centre (-371.8467, 0.508) ccw
  line L384 (-370.2603, 0) -> (-371.8467, 0)
  arc A191 (-370.2603, 0) -> (-369.7829, 0.3343) centre (-370.2603, 0.508) ccw
  line L385 (-367.8707, 5.588) -> (-369.7829, 0.3343)
  line L386 (-375.8504, 5.588) -> (-374.2363, 5.588)
  line L387 (-380.3037, 0.3343) -> (-382.2159, 5.588)
  line L388 (-387.0128, 0) -> (-379.0332, 0) construction
  line L389 (-383.83, 5.588) -> (-385.7422, 0.3343)
  arc A192 (-386.2196, 0) -> (-385.7422, 0.3343) centre (-386.2196, 0.508) ccw
  line L390 (-386.2196, 0) -> (-387.806, 0)
  arc A193 (-388.2834, 0.3343) -> (-387.806, 0) centre (-387.806, 0.508) ccw
  line L391 (-388.2834, 0.3343) -> (-390.1956, 5.588)
  arc A194 (-380.3037, 0.3343) -> (-379.8264, 0) centre (-379.8264, 0.508) ccw
  line L392 (-378.2399, 0) -> (-379.8264, 0)
  arc A195 (-378.2399, 0) -> (-377.7626, 0.3343) centre (-378.2399, 0.508) ccw
  line L393 (-375.8504, 5.588) -> (-377.7626, 0.3343)
  line L394 (-383.83, 5.588) -> (-382.2159, 5.588)
  line L395 (-388.2834, 0.3343) -> (-390.1956, 5.588)
  line L396 (-394.9924, 0) -> (-387.0128, 0) construction
  line L397 (-391.8097, 5.588) -> (-393.7219, 0.3343)
  arc A196 (-394.1992, 0) -> (-393.7219, 0.3343) centre (-394.1992, 0.508) ccw
  line L398 (-394.1992, 0) -> (-395.7857, 0)
  arc A197 (-396.263, 0.3343) -> (-395.7857, 0) centre (-395.7857, 0.508) ccw
  line L399 (-396.263, 0.3343) -> (-398.1752, 5.588)
  arc A198 (-388.2834, 0.3343) -> (-387.806, 0) centre (-387.806, 0.508) ccw
  line L400 (-386.2196, 0) -> (-387.806, 0)
  arc A199 (-386.2196, 0) -> (-385.7422, 0.3343) centre (-386.2196, 0.508) ccw
  line L401 (-383.83, 5.588) -> (-385.7422, 0.3343)
  line L402 (-391.8097, 5.588) -> (-390.1956, 5.588)
  line L403 (-396.263, 0.3343) -> (-398.1752, 5.588)
  line L404 (-402.9721, 0) -> (-394.9924, 0) construction
  line L405 (-399.7893, 5.588) -> (-401.7015, 0.3343)
  arc A200 (-402.1789, 0) -> (-401.7015, 0.3343) centre (-402.1789, 0.508) ccw
  line L406 (-402.1789, 0) -> (-403.7653, 0)
  arc A201 (-404.2427, 0.3343) -> (-403.7653, 0) centre (-403.7653, 0.508) ccw
  line L407 (-404.2427, 0.3343) -> (-406.1549, 5.588)
  arc A202 (-396.263, 0.3343) -> (-395.7857, 0) centre (-395.7857, 0.508) ccw
  line L408 (-394.1992, 0) -> (-395.7857, 0)
  arc A203 (-394.1992, 0) -> (-393.7219, 0.3343) centre (-394.1992, 0.508) ccw
  line L409 (-391.8097, 5.588) -> (-393.7219, 0.3343)
  line L410 (-399.7893, 5.588) -> (-398.1752, 5.588)
  line L411 (-404.2427, 0.3343) -> (-406.1549, 5.588)
  line L412 (-410.9517, 0) -> (-402.9721, 0) construction
  line L413 (-407.769, 5.588) -> (-409.6812, 0.3343)
  arc A204 (-410.1585, 0) -> (-409.6812, 0.3343) centre (-410.1585, 0.508) ccw
  line L414 (-410.1585, 0) -> (-411.7449, 0)
  arc A205 (-412.2223, 0.3343) -> (-411.7449, 0) centre (-411.7449, 0.508) ccw
  line L415 (-412.2223, 0.3343) -> (-414.1345, 5.588)
  arc A206 (-404.2427, 0.3343) -> (-403.7653, 0) centre (-403.7653, 0.508) ccw
  line L416 (-402.1789, 0) -> (-403.7653, 0)
  arc A207 (-402.1789, 0) -> (-401.7015, 0.3343) centre (-402.1789, 0.508) ccw
  line L417 (-399.7893, 5.588) -> (-401.7015, 0.3343)
  line L418 (-407.769, 5.588) -> (-406.1549, 5.588)
  line L419 (-412.2223, 0.3343) -> (-414.1345, 5.588)
  line L420 (-418.9314, 0) -> (-410.9517, 0) construction
  line L421 (-415.7486, 5.588) -> (-417.6608, 0.3343)
  arc A208 (-418.1382, 0) -> (-417.6608, 0.3343) centre (-418.1382, 0.508) ccw
  line L422 (-418.1382, 0) -> (-419.7246, 0)
  arc A209 (-420.202, 0.3343) -> (-419.7246, 0) centre (-419.7246, 0.508) ccw
  line L423 (-420.202, 0.3343) -> (-422.1142, 5.588)
  arc A210 (-412.2223, 0.3343) -> (-411.7449, 0) centre (-411.7449, 0.508) ccw
  line L424 (-410.1585, 0) -> (-411.7449, 0)
  arc A211 (-410.1585, 0) -> (-409.6812, 0.3343) centre (-410.1585, 0.508) ccw
  line L425 (-407.769, 5.588) -> (-409.6812, 0.3343)
  line L426 (-415.7486, 5.588) -> (-414.1345, 5.588)
  line L427 (-420.202, 0.3343) -> (-422.1142, 5.588)
  line L428 (-426.911, 0) -> (-418.9314, 0) construction
  line L429 (-423.7282, 5.588) -> (-425.6404, 0.3343)
  arc A212 (-426.1178, 0) -> (-425.6404, 0.3343) centre (-426.1178, 0.508) ccw
  line L430 (-426.1178, 0) -> (-427.7042, 0)
  arc A213 (-428.1816, 0.3343) -> (-427.7042, 0) centre (-427.7042, 0.508) ccw
  line L431 (-428.1816, 0.3343) -> (-430.0938, 5.588)
  arc A214 (-420.202, 0.3343) -> (-419.7246, 0) centre (-419.7246, 0.508) ccw
  line L432 (-418.1382, 0) -> (-419.7246, 0)
  arc A215 (-418.1382, 0) -> (-417.6608, 0.3343) centre (-418.1382, 0.508) ccw
  line L433 (-415.7486, 5.588) -> (-417.6608, 0.3343)
  line L434 (-423.7282, 5.588) -> (-422.1142, 5.588)
  line L435 (-428.1816, 0.3343) -> (-430.0938, 5.588)
  line L436 (-434.8907, 0) -> (-426.911, 0) construction
  line L437 (-431.7079, 5.588) -> (-433.6201, 0.3343)
  arc A216 (-434.0975, 0) -> (-433.6201, 0.3343) centre (-434.0975, 0.508) ccw
  line L438 (-434.0975, 0) -> (-435.6839, 0)
  arc A217 (-436.1612, 0.3343) -> (-435.6839, 0) centre (-435.6839, 0.508) ccw
  line L439 (-436.1612, 0.3343) -> (-438.0735, 5.588)
  arc A218 (-428.1816, 0.3343) -> (-427.7042, 0) centre (-427.7042, 0.508) ccw
  line L440 (-426.1178, 0) -> (-427.7042, 0)
  arc A219 (-426.1178, 0) -> (-425.6404, 0.3343) centre (-426.1178, 0.508) ccw
  line L441 (-423.7282, 5.588) -> (-425.6404, 0.3343)
  line L442 (-431.7079, 5.588) -> (-430.0938, 5.588)
  line L443 (-436.1612, 0.3343) -> (-438.0735, 5.588)
  line L444 (-442.8703, 0) -> (-434.8907, 0) construction
  line L445 (-439.6875, 5.588) -> (-441.5997, 0.3343)
  arc A220 (-442.0771, 0) -> (-441.5997, 0.3343) centre (-442.0771, 0.508) ccw
  line L446 (-442.0771, 0) -> (-443.6635, 0)
  arc A221 (-444.1409, 0.3343) -> (-443.6635, 0) centre (-443.6635, 0.508) ccw
  line L447 (-444.1409, 0.3343) -> (-446.0531, 5.588)
  arc A222 (-436.1612, 0.3343) -> (-435.6839, 0) centre (-435.6839, 0.508) ccw
  line L448 (-434.0975, 0) -> (-435.6839, 0)
  arc A223 (-434.0975, 0) -> (-433.6201, 0.3343) centre (-434.0975, 0.508) ccw
  line L449 (-431.7079, 5.588) -> (-433.6201, 0.3343)
  line L450 (-439.6875, 5.588) -> (-438.0735, 5.588)
  line L451 (-444.1409, 0.3343) -> (-446.0531, 5.588)
  line L452 (-450.85, 0) -> (-442.8703, 0) construction
  line L453 (-447.6672, 5.588) -> (-449.5794, 0.3343)
  arc A224 (-450.0567, 0) -> (-449.5794, 0.3343) centre (-450.0567, 0.508) ccw
  line L454 (-450.0567, 0) -> (-451.6432, 0)
  arc A225 (-452.1205, 0.3343) -> (-451.6432, 0) centre (-451.6432, 0.508) ccw
  line L455 (-452.1205, 0.3343) -> (-454.0327, 5.588)
  arc A226 (-444.1409, 0.3343) -> (-443.6635, 0) centre (-443.6635, 0.508) ccw
  line L456 (-442.0771, 0) -> (-443.6635, 0)
  arc A227 (-442.0771, 0) -> (-441.5997, 0.3343) centre (-442.0771, 0.508) ccw
  line L457 (-439.6875, 5.588) -> (-441.5997, 0.3343)
  line L458 (-447.6672, 5.588) -> (-446.0531, 5.588)
  line L459 (-452.1205, 0.3343) -> (-454.0327, 5.588)
  line L460 (-458.8296, 0) -> (-450.85, 0) construction
  line L461 (-455.6468, 5.588) -> (-457.559, 0.3343)
  arc A228 (-458.0364, 0) -> (-457.559, 0.3343) centre (-458.0364, 0.508) ccw
  line L462 (-458.0364, 0) -> (-459.6228, 0)
  arc A229 (-460.1002, 0.3343) -> (-459.6228, 0) centre (-459.6228, 0.508) ccw
  line L463 (-460.1002, 0.3343) -> (-462.0124, 5.588)
  arc A230 (-452.1205, 0.3343) -> (-451.6432, 0) centre (-451.6432, 0.508) ccw
  line L464 (-450.0567, 0) -> (-451.6432, 0)
  arc A231 (-450.0567, 0) -> (-449.5794, 0.3343) centre (-450.0567, 0.508) ccw
  line L465 (-447.6672, 5.588) -> (-449.5794, 0.3343)
  line L466 (-455.6468, 5.588) -> (-454.0327, 5.588)
  line L467 (-460.1002, 0.3343) -> (-462.0124, 5.588)
  line L468 (-466.8093, 0) -> (-458.8296, 0) construction
  line L469 (-463.6265, 5.588) -> (-465.5387, 0.3343)
  arc A232 (-466.016, 0) -> (-465.5387, 0.3343) centre (-466.016, 0.508) ccw
  line L470 (-466.016, 0) -> (-467.6025, 0)
  arc A233 (-468.0798, 0.3343) -> (-467.6025, 0) centre (-467.6025, 0.508) ccw
  line L471 (-468.0798, 0.3343) -> (-469.992, 5.588)
  arc A234 (-460.1002, 0.3343) -> (-459.6228, 0) centre (-459.6228, 0.508) ccw
  line L472 (-458.0364, 0) -> (-459.6228, 0)
  arc A235 (-458.0364, 0) -> (-457.559, 0.3343) centre (-458.0364, 0.508) ccw
  line L473 (-455.6468, 5.588) -> (-457.559, 0.3343)
  line L474 (-463.6265, 5.588) -> (-462.0124, 5.588)
  line L475 (-468.0798, 0.3343) -> (-469.992, 5.588)
  line L476 (-474.7889, 0) -> (-466.8093, 0) construction
  line L477 (-471.6061, 5.588) -> (-473.5183, 0.3343)
  arc A236 (-473.9957, 0) -> (-473.5183, 0.3343) centre (-473.9957, 0.508) ccw
  line L478 (-473.9957, 0) -> (-475.5821, 0)
  arc A237 (-476.0595, 0.3343) -> (-475.5821, 0) centre (-475.5821, 0.508) ccw
  line L479 (-476.0595, 0.3343) -> (-477.9717, 5.588)
  arc A238 (-468.0798, 0.3343) -> (-467.6025, 0) centre (-467.6025, 0.508) ccw
  line L480 (-466.016, 0) -> (-467.6025, 0)
  arc A239 (-466.016, 0) -> (-465.5387, 0.3343) centre (-466.016, 0.508) ccw
  line L481 (-463.6265, 5.588) -> (-465.5387, 0.3343)
  line L482 (-471.6061, 5.588) -> (-469.992, 5.588)
  line L483 (-476.0595, 0.3343) -> (-477.9717, 5.588)
  line L484 (-482.7685, 0) -> (-474.7889, 0) construction
  line L485 (-479.5858, 5.588) -> (-481.498, 0.3343)
  arc A240 (-481.9753, 0) -> (-481.498, 0.3343) centre (-481.9753, 0.508) ccw
  line L486 (-481.9753, 0) -> (-483.5618, 0)
  arc A241 (-484.0391, 0.3343) -> (-483.5618, 0) centre (-483.5618, 0.508) ccw
  line L487 (-484.0391, 0.3343) -> (-485.9513, 5.588)
  arc A242 (-476.0595, 0.3343) -> (-475.5821, 0) centre (-475.5821, 0.508) ccw
  line L488 (-473.9957, 0) -> (-475.5821, 0)
  arc A243 (-473.9957, 0) -> (-473.5183, 0.3343) centre (-473.9957, 0.508) ccw
  line L489 (-471.6061, 5.588) -> (-473.5183, 0.3343)
  line L490 (-479.5858, 5.588) -> (-477.9717, 5.588)
  line L491 (-484.0391, 0.3343) -> (-485.9513, 5.588)
  line L492 (-490.7482, 0) -> (-482.7685, 0) construction
  line L493 (-487.5654, 5.588) -> (-489.4776, 0.3343)
  arc A244 (-489.955, 0) -> (-489.4776, 0.3343) centre (-489.955, 0.508) ccw
  line L494 (-489.955, 0) -> (-491.5414, 0)
  arc A245 (-492.0188, 0.3343) -> (-491.5414, 0) centre (-491.5414, 0.508) ccw
  line L495 (-492.0188, 0.3343) -> (-493.931, 5.588)
  arc A246 (-484.0391, 0.3343) -> (-483.5618, 0) centre (-483.5618, 0.508) ccw
  line L496 (-481.9753, 0) -> (-483.5618, 0)
  arc A247 (-481.9753, 0) -> (-481.498, 0.3343) centre (-481.9753, 0.508) ccw
  line L497 (-479.5858, 5.588) -> (-481.498, 0.3343)
  line L498 (-487.5654, 5.588) -> (-485.9513, 5.588)
  line L499 (-492.0188, 0.3343) -> (-493.931, 5.588)
  line L500 (-498.7278, 0) -> (-490.7482, 0) construction
  line L501 (-495.545, 5.588) -> (-497.4573, 0.3343)
  arc A248 (-497.9346, 0) -> (-497.4573, 0.3343) centre (-497.9346, 0.508) ccw
  line L502 (-497.9346, 0) -> (-499.521, 0)
  arc A249 (-499.9984, 0.3343) -> (-499.521, 0) centre (-499.521, 0.508) ccw
  line L503 (-499.9984, 0.3343) -> (-501.9106, 5.588)
  arc A250 (-492.0188, 0.3343) -> (-491.5414, 0) centre (-491.5414, 0.508) ccw
  line L504 (-489.955, 0) -> (-491.5414, 0)
  arc A251 (-489.955, 0) -> (-489.4776, 0.3343) centre (-489.955, 0.508) ccw
  line L505 (-487.5654, 5.588) -> (-489.4776, 0.3343)
  line L506 (-495.545, 5.588) -> (-493.931, 5.588)
  line L507 (-499.9984, 0.3343) -> (-501.9106, 5.588)
  line L508 (-506.7075, 0) -> (-498.7278, 0) construction
  line L509 (-503.5247, 5.588) -> (-505.4369, 0.3343)
  arc A252 (-505.9143, 0) -> (-505.4369, 0.3343) centre (-505.9143, 0.508) ccw
  line L510 (-505.9143, 0) -> (-507.5007, 0)
  arc A253 (-507.9781, 0.3343) -> (-507.5007, 0) centre (-507.5007, 0.508) ccw
  line L511 (-507.9781, 0.3343) -> (-509.8903, 5.588)
  arc A254 (-499.9984, 0.3343) -> (-499.521, 0) centre (-499.521, 0.508) ccw
  line L512 (-497.9346, 0) -> (-499.521, 0)
  arc A255 (-497.9346, 0) -> (-497.4573, 0.3343) centre (-497.9346, 0.508) ccw
  line L513 (-495.545, 5.588) -> (-497.4573, 0.3343)
  line L514 (-503.5247, 5.588) -> (-501.9106, 5.588)
  line L515 (-507.9781, 0.3343) -> (-509.8903, 5.588)
  line L516 (-514.6871, 0) -> (-506.7075, 0) construction
  line L517 (-511.5043, 5.588) -> (-513.4165, 0.3343)
  arc A256 (-513.8939, 0) -> (-513.4165, 0.3343) centre (-513.8939, 0.508) ccw
  line L518 (-513.8939, 0) -> (-515.4803, 0)
  arc A257 (-515.9577, 0.3343) -> (-515.4803, 0) centre (-515.4803, 0.508) ccw
  line L519 (-515.9577, 0.3343) -> (-517.8699, 5.588)
  arc A258 (-507.9781, 0.3343) -> (-507.5007, 0) centre (-507.5007, 0.508) ccw
  line L520 (-505.9143, 0) -> (-507.5007, 0)
  arc A259 (-505.9143, 0) -> (-505.4369, 0.3343) centre (-505.9143, 0.508) ccw
  line L521 (-503.5247, 5.588) -> (-505.4369, 0.3343)
  line L522 (-511.5043, 5.588) -> (-509.8903, 5.588)
  line L523 (-515.9577, 0.3343) -> (-517.8699, 5.588)
  line L524 (-522.6668, 0) -> (-514.6871, 0) construction
  line L525 (-519.484, 5.588) -> (-521.3962, 0.3343)
  arc A260 (-521.8736, 0) -> (-521.3962, 0.3343) centre (-521.8736, 0.508) ccw
  line L526 (-521.8736, 0) -> (-523.46, 0)
  arc A261 (-523.9373, 0.3343) -> (-523.46, 0) centre (-523.46, 0.508) ccw
  line L527 (-523.9373, 0.3343) -> (-525.8496, 5.588)
  arc A262 (-515.9577, 0.3343) -> (-515.4803, 0) centre (-515.4803, 0.508) ccw
  line L528 (-513.8939, 0) -> (-515.4803, 0)
  arc A263 (-513.8939, 0) -> (-513.4165, 0.3343) centre (-513.8939, 0.508) ccw
  line L529 (-511.5043, 5.588) -> (-513.4165, 0.3343)
  line L530 (-519.484, 5.588) -> (-517.8699, 5.588)
  line L531 (-523.9373, 0.3343) -> (-525.8496, 5.588)
  line L532 (-530.6464, 0) -> (-522.6668, 0) construction
  line L533 (-527.4636, 5.588) -> (-529.3758, 0.3343)
  arc A264 (-529.8532, 0) -> (-529.3758, 0.3343) centre (-529.8532, 0.508) ccw
  line L534 (-529.8532, 0) -> (-531.4396, 0)
  arc A265 (-531.917, 0.3343) -> (-531.4396, 0) centre (-531.4396, 0.508) ccw
  line L535 (-531.917, 0.3343) -> (-533.8292, 5.588)
  arc A266 (-523.9373, 0.3343) -> (-523.46, 0) centre (-523.46, 0.508) ccw
  line L536 (-521.8736, 0) -> (-523.46, 0)
  arc A267 (-521.8736, 0) -> (-521.3962, 0.3343) centre (-521.8736, 0.508) ccw
  line L537 (-519.484, 5.588) -> (-521.3962, 0.3343)
  line L538 (-527.4636, 5.588) -> (-525.8496, 5.588)
  line L539 (-531.917, 0.3343) -> (-533.8292, 5.588)
  line L540 (-538.6261, 0) -> (-530.6464, 0) construction
  line L541 (-535.4433, 5.588) -> (-537.3555, 0.3343)
  arc A268 (-537.8328, 0) -> (-537.3555, 0.3343) centre (-537.8328, 0.508) ccw
  line L542 (-537.8328, 0) -> (-539.4193, 0)
  arc A269 (-539.8966, 0.3343) -> (-539.4193, 0) centre (-539.4193, 0.508) ccw
  line L543 (-539.8966, 0.3343) -> (-541.8088, 5.588)
  arc A270 (-531.917, 0.3343) -> (-531.4396, 0) centre (-531.4396, 0.508) ccw
  line L544 (-529.8532, 0) -> (-531.4396, 0)
  arc A271 (-529.8532, 0) -> (-529.3758, 0.3343) centre (-529.8532, 0.508) ccw
  line L545 (-527.4636, 5.588) -> (-529.3758, 0.3343)
  line L546 (-535.4433, 5.588) -> (-533.8292, 5.588)
  line L547 (-539.8966, 0.3343) -> (-541.8088, 5.588)
  line L548 (-546.6057, 0) -> (-538.6261, 0) construction